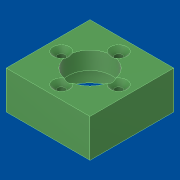
# Autodesk Inventor part: 402-gearbox-housing
Saved by Autodesk Inventor 2018 (Build 220112000, 112)
## iProperties
Created: 2020-06-11
Part Number: 402-gearbox-housing
Material: Generic
Document SubType Name: Modeling
Designer: Bunny320
Density: 1 g/cm^3
Appearance: Smooth - Dark Forest Green
Author: Bunny320
## iProperties of the stored document 402-gearbox-housing-dummy_3DPrint.ipt
Created: 2020-06-12
Part Number: 402-gearbox-housing-dummy_3DPrint
Material: Generic
Document SubType Name: Modeling
Designer: Bunny320
Density: 1 g/cm^3
Appearance: Default
Author: Bunny320
Autodesk Inventor part; units mm, degrees
ref_plane "YZ Plane" through (0, 0, 0) normal (1, 0, 0) x (0, 1, 0)
ref_plane "XZ Plane" through (0, 0, 0) normal (0, 1, 0) x (-1, 0, 0)
ref_plane "XY Plane" through (0, 0, 0) normal (0, 0, 1) x (1, 0, 0)
sketch "Sketch1" plane through (0, 0, 0) normal (0, 0, 1) x (1, 0, 0)
  line L0 (-19, -19) -> (19, -19)
  line L1 (19, -19) -> (19, 19)
  line L2 (19, 19) -> (-19, 19)
  line L3 (-19, 19) -> (-19, -19)
  line L4 (-19, -19) -> (19, 19) construction
  line L5 (19, -19) -> (-19, 19) construction
  point P0 (0, 0)
  dimension "d0" = 38
  constraints: 12 end point, 2 midpoint, 2 parallel, 2 perpendicular, 1 horizontal
  measures "d0" distance of L1.end L2.end
extrude "Extrusion1" add sketch "Sketch1" along normal blind 100
sketch "Sketch2" plane through (0, 0, 0) normal (0, 0, -1) x (-1, 0, 0)
  circle A0 centre (0, 0) radius 16.15
  dimension "d3" = 32.3
  constraints: 1 centre point, 1 coincident
  measures "d3" diameter of A0
extrude "Extrusion2" cut sketch "Sketch2" against normal blind 32
sketch "Sketch3" plane through (0, 0, 100) normal (0, 0, 1) x (1, 0, 0)
  circle A0 centre (0, 0) radius 17
  dimension "d6" = 34
  constraints: 1 centre point, 1 coincident
  measures "d6" diameter of A0
extrude "Extrusion3" cut sketch "Sketch3" against normal blind 60
sketch "Sketch4" plane through (0, 0, 40) normal (0, 0, 1) x (1, 0, 0)
  circle A0 centre (0, 0) radius 10
  dimension "d9" = 20
  constraints: 1 centre point, 1 coincident
  measures "d9" diameter of A0
extrude "Extrusion4" cut sketch "Sketch4" against normal through all
sketch "Sketch5" plane through (0, 0, 40) normal (0, 0, 1) x (1, 0, 0)
  point P0 (0, 0)
  point P1 (0, 13)
  dimension "d12" = 13
  constraints: 1 vertical alignment
  measures "d12" distance of point (0, 0) point (0, 13)
hole "Hole1" at (0, 13, 40) direction (0, 0, -1) diameter 3.4 end through all countersink diameter 7.5 countersink angle 90 clearance for "Countersunk Flat Head Hex Socket Screw DIN EN ISO 10642" size "M3" standard "DIN"
pattern_circular "Circular Pattern1" count 4 over 360 about axis through (0, 0, -10) along (0, 0, 1) of "Hole1"
sketch "Sketch6" plane through (0, 0, 100) normal (0, 0, 1) x (1, 0, 0)
  line L0 (26.1087, -24.9255) -> (-24.3734, -24.9255)
  line L1 (-24.3734, -24.9255) -> (-24.3734, 25.8721)
  line L2 (-24.3734, 25.8721) -> (26.1087, 25.8721)
  line L3 (26.1087, 25.8721) -> (26.1087, -24.9255)
  point P0 (0, 0)
  constraints: 8 end point, 2 parallel, 1 horizontal, 1 perpendicular
extrude "Extrusion5" cut sketch "Sketch6" against normal up to surface (60 mm away)
sketch "Sketch7" plane through (0, 0, 0) normal (0, 0, -1) x (-1, 0, 0)
  line L0 (21.4324, -23.2888) -> (-21.2074, -23.2888)
  line L1 (-21.2074, -23.2888) -> (-21.2074, 21.7137)
  line L2 (-21.2074, 21.7137) -> (21.4324, 21.7137)
  line L3 (21.4324, 21.7137) -> (21.4324, -23.2888)
  point P0 (0, 0)
  constraints: 8 end point, 2 parallel, 1 horizontal, 1 perpendicular
extrude "Extrusion6" cut sketch "Sketch7" against normal blind 22.75
body "Solid1"
